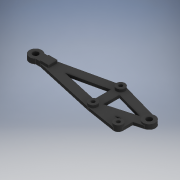
# Autodesk Inventor part: RAMPS Mount
Saved by Autodesk Inventor 2020.2 (Build 242310000, 310)
## iProperties
Created: 2019-12-18
Part Number: RAMPS Mount
Material: ABS Plastic
Document SubType Name: Modeling
Designer: Richard Hall
Density: 1.06 g/cm^3
Appearance: Rubber - Black
Author: Richard Hall
Autodesk Inventor part; units mm, degrees
ref_plane "YZ Plane" through (0, 0, 0) normal (1, 0, 0) x (0, 1, 0)
ref_plane "XZ Plane" through (0, 0, 0) normal (0, 1, 0) x (-1, 0, 0)
ref_plane "XY Plane" through (0, 0, 0) normal (0, 0, 1) x (1, 0, 0)
sketch "Sketch1" plane through (0, 0, 0) normal (0, 1, 0) x (-1, 0, 0)
  circle A0 centre (0, 0) radius 6.325
  circle A1 centre (-118.053, 0) radius 6.325
  circle A2 centre (-74.04, -14.35) radius 4.5
  circle A3 centre (-74.04, 14.35) radius 4.5
  circle A4 centre (-105.29, 19.35) radius 4.5
  line L0 (-4.4447, 4.5) -> (-9.5157, 4.5)
  line L1 (-9.5157, 4.5) -> (-73.0558, 18.7411)
  line L2 (-73.329, 18.7935) -> (-104.579, 23.7935)
  line L3 (-119.775, -6.0861) -> (-75.2652, -18.68)
  line L4 (-75.2652, 18.68) -> (-119.775, 6.0861)
  line L5 (-109.79, 19.35) -> (-109.79, 8.9113)
  line L6 (-69.54, 14.35) -> (-69.54, -14.35)
  line L7 (-78.54, 14.35) -> (-78.54, -14.35)
  line L8 (-108.8889, 0) -> (-78.54, 8.5871)
  line L9 (-108.8889, 0) -> (-78.54, -8.5871)
  line L10 (-4.4447, -4.5) -> (-9.5157, -4.5)
  line L11 (-9.5157, -4.5) -> (-73.0558, -18.7411)
  line L12 (-69.54, 8.9143) -> (-29.7668, 0)
  line L13 (-29.7668, 0) -> (-69.54, -8.9143)
  line L14 (-106.001, 14.9065) -> (-74.751, 9.9065)
  line L15 (-100.79, 19.35) -> (-100.79, 11.4578)
  point P0 (-94.8865, 13.1282)
  point P1 (-100.79, 14.0728)
  dimension "d0" = 12.65
  dimension "d1" = 12.65
  dimension "d2" = 9
  dimension "d3" = 9
  dimension "d4" = 9
  dimension "d5" = 28.7
  dimension "d6" = 14.35
  dimension "d7" = 31.25
  dimension "d8" = 5
  dimension "d9" = 74.04
  dimension "d10" = 118.053
  dimension "d11" = 5.071
  dimension "d12" = 8.82
  dimension "d13" = 8.82
  dimension "d14" = 9
  dimension "d15" = 8.82
  constraints: 32 end point, 18 point on circle, 14 tangent, 6 point on line, 5 centre point, 5 parallel, 4 vertical, 2 horizontal, 2 horizontal alignment, 2 vertical alignment, 1 coincident
  measures "d0" diameter of A0
  measures "d1" diameter of A1
  measures "d2" diameter of A2
  measures "d3" diameter of A3
  measures "d4" diameter of A4
  measures "d5" distance of A2.centre A3.centre
  measures "d6" vertical distance of A3.centre point (0, 0)
  measures "d7" horizontal distance of A4.centre A3.centre
  measures "d8" vertical distance of A4.centre A3.centre
  measures "d9" horizontal distance of A2.centre point (0, 0)
  measures "d10" distance of point (0, 0) A1.centre
  measures "d11" distance of L0.start L0.end
  measures "d12" distance between parallel lines of L3 L9
  measures "d13" distance between parallel lines of L4 L8
  measures "d14" distance between parallel lines of L10 L0
  measures "d15" distance between parallel lines of L1 L12
extrude "Extrusion1" add sketch "Sketch1" along normal blind 3 contours A0 | A0 L10 L11 A2 L6 L13 L12 A3 L1 L0 | A3 | A2 | L6 A2 L7 L14 A3 | A3 L4 L14 L15 A4 L2 | L3 A1 L4 L14 L7 L8 L9 A2 | L14 L7 A3 | A3 L7 L14 L4 | A4 | A1 | L15 L14 A4 | A4 L14 L15 L4 L5
sketch "Sketch2" plane through (0, 3, 0) normal (0, 1, 0) x (1, 0, 0)
  arc A0 (73.0558, -18.7411) -> (73.329, -18.7935) centre (74.04, -14.35) ccw projected
  circle A1 centre (74.04, -14.35) radius 4.5
  arc A2 (75.2652, 18.68) -> (73.0558, 18.7411) centre (74.04, 14.35) ccw projected
  arc A3 (104.579, -23.7935) -> (109.79, -19.35) centre (105.29, -19.35) ccw projected
  circle A4 centre (105.29, -19.35) radius 4.5
  circle A5 centre (74.04, 14.35) radius 4.5
  point P0 (0, 0)
  point P1 (109.79, -19.35)
  point P2 (73.0558, -18.7411)
  point P3 (75.2652, 18.68)
  constraints: 3 centre point, 3 coincident, 3 concentric
extrude "Extrusion2" add sketch "Sketch2" along normal blind 3
sketch "Sketch3" plane through (0, 3, 0) normal (0, 1, 0) x (1, 0, 0)
  arc A0 (119.775, -6.0861) -> (119.775, 6.0861) centre (118.053, 0) ccw projected
  circle A1 centre (118.053, 0) radius 6.325
  circle A2 centre (0, 0) radius 6.325
  arc A3 (4.4447, 4.5) -> (4.4447, -4.5) centre (0, 0) ccw projected
  line L0 (4.4447, -4.5) -> (18.04, -4.5)
  line L1 (18.04, -4.5) -> (18.04, 4.5)
  line L2 (18.04, 4.5) -> (4.4447, 4.5)
  line L3 (4.4447, 4.5) -> (4.4447, -4.5) construction
  point P0 (119.775, 6.0861)
  point P1 (119.775, -6.0861)
  dimension "d20" = 9
  dimension "d21" = 18.04
  constraints: 8 end point, 2 centre point, 2 coincident, 2 concentric, 2 parallel, 2 point on circle, 1 horizontal, 1 perpendicular
  measures "d20" distance of L2.end L0.start
  measures "d21" distance from line of L1 point (0, 0)
extrude "Extrusion3" add sketch "Sketch3" along normal blind 2
sketch "Sketch4" plane through (0, 5, 0) normal (0, 1, 0) x (1, 0, 0)
  line L0 (18.04, 4.5) -> (4.4447, 4.5) projected
  arc A0 (4.4447, 4.5) -> (4.4447, -4.5) centre (0, 0) ccw projected
  line L1 (4.4447, -4.5) -> (18.04, -4.5) projected
  line L2 (18.04, -4.5) -> (18.04, 4.5) projected
  line L3 (18.04, 4.5) -> (18.04, -4.5) projected
  line L4 (18.04, -4.5) -> (9.04, -4.5)
  line L5 (9.04, -4.5) -> (9.04, 4.5)
  line L6 (9.04, 4.5) -> (18.04, 4.5)
  line L7 (18.04, 4.5) -> (18.04, -4.5)
  dimension "d24" = 9
  dimension "d25" = 9
  constraints: 8 end point, 2 parallel, 1 horizontal, 1 perpendicular
  measures "d24" distance of L5.end L6.end
  measures "d25" distance of L4.end L5.end
extrude "Extrusion4" add sketch "Sketch4" along normal blind 1 contours L2 L1 L5 L0
sketch "Sketch5" plane through (0, 5, 0) normal (0, 1, 0) x (1, 0, 0)
  arc A0 (4.4447, 4.5) -> (4.4447, -4.5) centre (0, 0) ccw projected
  circle A1 centre (118.053, 0) radius 6.325 projected
  constraints: 2 coincident
hole "Hole1" at (0, 5, 0) at (118.053, 5, 0) direction (0, -1, 0) diameter 6 end through all
sketch "Sketch6" plane through (74.04, 6, -14.35) normal (0, 1, 0) x (1, 0, 0)
  circle A0 centre (0, 0) radius 4.5 projected
  circle A1 centre (0, -28.7) radius 4.5 projected
  circle A2 centre (31.25, -33.7) radius 4.5 projected
  point P0 (-74.04, -14.35)
  constraints: 3 coincident
hole "Hole2" at (74.04, 6, -14.35) at (74.04, 6, 14.35) at (105.29, 6, 19.35) direction (0, -1, 0) diameter 4 end through all
equation "\"d0\" = d1"
equation "\"d2\" = d3"
equation "\"d3\" = d4"
equation "\"d6\" = 0.5 * d5"
equation "\"d13\" = d12"
equation "\"d15\" = d12"
body "Solid1"
